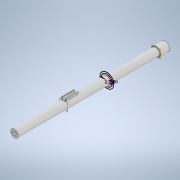
# Autodesk Inventor part: Blow Dart
Saved by Autodesk Inventor 2021 (Build 250183000, 183)
## iProperties
Created: 2020-06-11
Part Number: Blow Dart
Material: Generic
Document SubType Name: Modeling
Designer: saipr
Density: 1 g/cm^3
Appearance: Default
Author: saipr
Autodesk Inventor part; units mm, degrees
ref_plane "YZ Plane" through (0, 0, 0) normal (1, 0, 0) x (0, 1, 0)
ref_plane "XZ Plane" through (0, 0, 0) normal (0, 1, 0) x (-1, 0, 0)
ref_plane "XY Plane" through (0, 0, 0) normal (0, 0, 1) x (1, 0, 0)
sketch "Sketch1" plane through (0, 0, 0) normal (0, 0, 1) x (1, 0, 0)
  circle A0 centre (0, 0) radius 6.985
  circle A1 centre (0, 0) radius 15.875
  dimension "d0" = 13.97
  dimension "d1" = 31.75
  constraints: 2 centre point, 2 coincident
  measures "d0" diameter of A0
  measures "d1" diameter of A1
extrude "Extrusion1" add sketch "Sketch1" along normal blind 609.6
ref_plane "Work Plane1" through (0, 0, 25.4) normal (0, 0, -1) x (-1, 0, 0)
sketch "Sketch2" plane through (0, 0, 25.4) normal (0, 0, -1) x (-1, 0, 0)
  circle A0 centre (0, 0) radius 19.05
  circle A1 centre (0, 0) radius 15.875
  dimension "d5" = 38.1
  constraints: 2 centre point, 2 coincident
  measures "d5" diameter of A0
extrude "Extrusion2" add sketch "Sketch2" along normal blind 38.1
ref_plane "Work Plane2" through (0, 0, 406.4) normal (0, 0, -1) x (-1, 0, 0)
sketch "Sketch4" plane through (0, 0, 406.4) normal (0, 0, -1) x (-1, 0, 0)
  circle A0 centre (0, 0) radius 15.875 projected
  arc A1 (-5.5104, 25.3806) -> (5.5104, 25.3806) centre (0, 22.225) ccw
  line L0 (8.9871, 25.3806) -> (5.5104, 25.3806)
  line L1 (-5.5104, 25.3806) -> (-8.9871, 25.3806)
  arc A2 (-8.9871, 25.3806) -> (-5.8921, 14.7411) centre (0, 22.225) ccw
  arc A3 (5.8921, 14.7411) -> (8.9871, 25.3806) centre (0, 22.225) ccw
  line L2 (5.8921, 14.7411) -> (-5.8921, 14.7411)
  point P0 (0, 15.875)
  constraints: 8 point on circle, 6 end point, 3 centre point, 3 horizontal, 1 coincident
extrude "Extrusion3" add sketch "Sketch4" along normal blind 50.8 contours A0 A1 L0 A3 | A2 L1 A1 A0
ref_plane "Work Plane4" through (0, 0, 228.6) normal (0, 0, -1) x (-1, 0, 0)
sketch "Sketch6" plane through (0, 0, 228.6) normal (0, 0, -1) x (-1, 0, 0)
  circle A0 centre (0, 0) radius 15.875
  circle A1 centre (0, 0) radius 28.575
  circle A2 centre (0, 0) radius 22.225
  circle A3 centre (-22.225, 0) radius 6.35
  dimension "d23" = 44.45
  dimension "d22" = 57.15
  dimension "d24" = 12.7
  constraints: 3 centre point, 3 coincident, 1 horizontal alignment, 2 other
  measures "d22" diameter of A1
  measures "d24" diameter of A3
body "Solid1"
